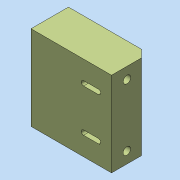
# Autodesk Inventor part: BC-10018
Saved by Autodesk Inventor 2016 (Build 200138000, 138)
## iProperties
Created: 2015-09-15
Part Number: BC-10018
Project: Xxxxxxxxxx xxxxxxxxx XXX
Cost Center: 0.00.00.000
Material: Aço Carbono
Document SubType Name: Modeling
Designer: Reinaldo.Basílio
Mass: 36242.3 g
Surface Area: 2210.86 cm^2
Volume: 4605.12 cm^3
Density: 7.87 g/cm^3
Appearance: Zinc Chromate 2
RuleStatus: InUse
AfterMaterialChange0: file://_iMaterial
AfterAnyiPropertyChange0: file://_iMaterial
AfterDocNew0: file://_Naming_par
AfterDocNew1: file://_NameStart
AfterDocNew2: file://_NameStart1
AfterDocNew3: file://_Materiais
DocNumber: XXXXX-XXX-XXXX-00-001.ipt
Folder: .
Title: SSD
Author: Reinaldo.Basílio
Autodesk Inventor part; units mm, degrees
ref_plane "YZ Plane" through (0, 0, 0) normal (1, 0, 0) x (0, 1, 0)
ref_plane "XZ Plane" through (0, 0, 0) normal (0, 1, 0) x (-1, 0, 0)
ref_plane "XY Plane" through (0, 0, 0) normal (0, 0, 1) x (1, 0, 0)
sketch "Sketch5" plane through (0, 0, 0) normal (0, 1, 0) x (-1, 0, 0)
  line L0 (50, 113) -> (-50, 113)
  line L1 (-50, 113) -> (-50, -113)
  line L2 (-50, -113) -> (50, -113)
  line L3 (50, -113) -> (50, 113)
  point P0 (0, 0)
  point P1 (50, 0)
  point P2 (0, 113)
  dimension "d8" = 100
  dimension "d9" = 226
  constraints: 8 end point, 2 midpoint, 2 parallel, 1 horizontal, 1 horizontal alignment, 1 perpendicular, 1 vertical alignment
  measures "d8" distance of L0.start L0.end
  measures "d9" distance of L0.end L1.end
extrude "Extrusion5" add sketch "Sketch5" along normal blind 215
sketch "Sketch9" plane through (-50, 0, -113) normal (-1, 0, 0) x (0, 0, 1)
  line L0 (0, 215) -> (226, 215) projected
  line L1 (170, 180.25) -> (170, 140.25) construction
  line L2 (163.75, 180.25) -> (163.75, 140.25)
  line L3 (176.25, 140.25) -> (176.25, 180.25)
  arc A0 (176.25, 180.25) -> (163.75, 180.25) centre (170, 180.25) ccw
  arc A1 (163.75, 140.25) -> (176.25, 140.25) centre (170, 140.25) ccw
  line L4 (113, 215) -> (113, 186.8149) construction
  line L5 (56, 180.25) -> (56, 140.25) construction
  line L6 (62.25, 180.25) -> (62.25, 140.25)
  line L7 (49.75, 140.25) -> (49.75, 180.25)
  arc A2 (62.25, 180.25) -> (49.75, 180.25) centre (56, 180.25) ccw
  arc A3 (49.75, 140.25) -> (62.25, 140.25) centre (56, 140.25) ccw
  line L8 (180, 140.25) -> (180, 180.25)
  arc A4 (180, 180.25) -> (160, 180.25) centre (170, 180.25) ccw
  line L9 (160, 180.25) -> (160, 140.25)
  arc A5 (160, 140.25) -> (180, 140.25) centre (170, 140.25) ccw
  line L10 (46, 140.25) -> (46, 180.25)
  arc A6 (66, 180.25) -> (46, 180.25) centre (56, 180.25) ccw
  line L11 (66, 180.25) -> (66, 140.25)
  arc A7 (46, 140.25) -> (66, 140.25) centre (56, 140.25) ccw
  point P0 (113, 0)
  point P1 (170, 160.25)
  point P2 (56, 160.25)
  dimension "d41" = 34.75
  dimension "d42" = 40
  dimension "d44" = 114
  dimension "d45" = 57
  dimension "d46" = 12.5
  dimension "d47" = 20
  constraints: 26 end point, 16 point on circle, 11 symmetric about line, 8 centre point, 4 tangent, 2 midpoint, 2 parallel, 1 perpendicular, 1 vertical, 7 other
  measures "d41" distance from line of L1.start L0
  measures "d42" distance of L1.start L1.end
  measures "d44" distance between parallel lines of L5 L1
  measures "d45" distance between parallel lines of L4 L1
  measures "d46" distance between parallel lines of L2 L3
  measures "d47" distance between parallel lines of L9 L8
extrude "Extrusion7" cut sketch "Sketch9" against normal through all contours A0 L3 A1 L2 | L6 A3 L7 A2
extrude "Extrusion8" cut sketch "Sketch9" against normal blind 60
chamfer "Chamfer4" distance 20 angle 45 1 edges at (-50, 215, 0)
sketch "Sketch10" plane through (0, 215, 0) normal (0, 1, 0) x (1, 0, 0)
  circle A0 centre (8.7673, -82.5) radius 6
  circle A1 centre (9.1389, 82.5) radius 6
  circle A2 centre (8.7673, -82.5) radius 10
  circle A3 centre (9.1389, 82.5) radius 10
  point P0 (0, 0)
  dimension "d55" = 165
  dimension "d56" = 82.5
  dimension "d57" = 12
  dimension "d58" = 20
  constraints: 4 centre point, 2 equal radius
  measures "d55" vertical distance of A1.centre A0.centre
  measures "d56" vertical distance of A0.centre point (0, 0)
  measures "d57" diameter of A0
  measures "d58" diameter of A2
hole "Hole2" at (8.7673, 215, 82.5) at (9.1389, 215, -82.5) direction (0, -1, 0) diameter 20 depth 140
sketch "Sketch11" plane through (9.1389, 75, -82.5) normal (0, 1, 0) x (1, 0, 0)
  circle A0 centre (0, 0) radius 10 projected
  circle A1 centre (0, 0) radius 6
  circle A2 centre (-0.3716, -165) radius 6
  circle A3 centre (-0.3716, -165) radius 10 projected
  circle A4 centre (0, 0) radius 10 projected
  point P0 (-9.1389, -82.5)
  dimension "d66" = 12
  constraints: 2 centre point, 2 concentric, 1 coincident, 1 equal radius
  measures "d66" diameter of A1
hole "Hole3" at (9.1389, 75, -82.5) at (8.7673, 75, 82.5) direction (0, -1, 0) diameter 10.106 end through all thread size "M12x1.75" class "6H" standard "ISO Metric profile"
equation "\"d56\" = 0.5 * d55"
body "Solid5"
